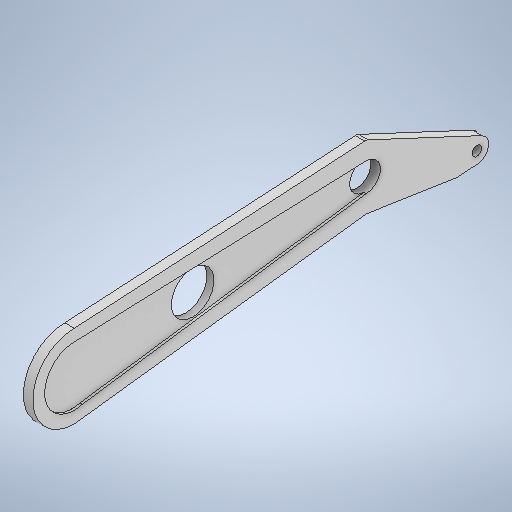
# Autodesk Inventor part: LINK1
Saved by Autodesk Inventor 2025 (Build 290162000, 162)
## iProperties
Created: 2026-05-21
Part Number: LINK1
Material: Generic
Document SubType Name: Sheet Metal
Designer: MSI
Density: 1 g/cm^3
Sheet Metal Rule: Default_mm
Appearance: Default
Author: MSI
Autodesk Inventor part; units mm, degrees
ref_plane "YZ Plane" through (0, 0, 0) normal (1, 0, 0) x (0, 1, 0)
ref_plane "XZ Plane" through (0, 0, 0) normal (0, 1, 0) x (-1, 0, 0)
ref_plane "XY Plane" through (0, 0, 0) normal (0, 0, 1) x (1, 0, 0)
sketch "Sketch1" plane through (0, 0, 0) normal (1, 0, 0) x (0, 1, 0)
  circle A0 centre (-2.6054, -169.98) radius 2.05
  arc A1 (17.5, -0.0099) -> (-16.9792, -4.2375) centre (0, 0) ccw
  arc A2 (-7.5969, -170.2704) -> (1.9242, -172.0973) centre (-2.6054, -169.98) ccw
  line L0 (17.5, -0.0099) -> (47.8897, -0.0099) construction
  line L1 (17.5, -0.0099) -> (24.6336, -122.6611)
  line L2 (24.3565, -124.1056) -> (1.9242, -172.0973)
  line L3 (-17.5, -0.0032) -> (-2.3777, -122.9531)
  line L4 (-2.3898, -123.7729) -> (-8.122, -161.2434)
  line L5 (-17.5, -0.0032) -> (-17.3824, -2.0256)
  line L6 (-8.122, -161.2434) -> (-7.5969, -170.2704)
  arc A3 (24.3565, -124.1056) -> (24.6336, -122.6611) centre (21.6387, -122.8353) ccw
  arc A4 (-2.3898, -123.7729) -> (-2.3777, -122.9531) centre (-5.3553, -123.3193) ccw
  circle A5 centre (4.5959, -51.0056) radius 9
  circle A6 centre (11.1072, -123.2673) radius 6
  circle A7 centre (0, 0) radius 12.5
  line L7 (12.5, 0) -> (17.103, -123.043)
  line L8 (-12.5, 0) -> (5.1072, -123.2673)
  point P0 (-2.3556, -123.3634)
  point P1 (24.5849, -123.4006)
  point P2 (-12.0001, -3.4995)
  dimension "d8" = 10
  dimension "d9" = 35
  dimension "d10" = 4.1
  dimension "d11" = 170
  dimension "d12" = 3
  dimension "d13" = 3
  dimension "d16" = 18
  dimension "d17" = 12
  dimension "d19" = 25
  constraints: 18 end point, 16 point on circle, 8 centre point, 8 tangent, 3 coincident, 2 parallel, 1 horizontal, 1 point on line
  measures "d8" diameter of A2
  measures "d9" diameter of A1
  measures "d10" diameter of A0
  measures "d11" distance of A0.centre point (0, 0)
  measures "d12" radius of A3
  measures "d13" radius of A4
  measures "d16" diameter of A5
  measures "d17" diameter of A6
  measures "d19" diameter of A7
extrude "Extrusion1" add sketch "Sketch1" along normal blind 4 contours L1 A3 L2 A2 L6 L4 A4 L3 A1
extrude "Extrusion2" add sketch "Sketch1" along normal blind 3 contours A6 L8 A7 L7
extrude "Extrusion3" add sketch "Sketch1" along normal blind 3 contours A7 L8 picked at (2.216, 2.7519)
equation "\"BendRadius\" = Thickness"
equation "\"BendReliefWidth\" = Thickness"
equation "\"BendReliefDepth\" = 0.5 * Thickness"
equation "\"CornerReliefSize\" = 4 * Thickness"
equation "\"MinimumRemnant\" = 2 * Thickness"
equation "\"TransitionRadius\" = BendRadius"
equation "\"JacobiRadiusSize\" = BendRadius"
equation "\"GapSize\" = Thickness"
equation "\"Thickness\" = 0.5"
body "Solid1"
